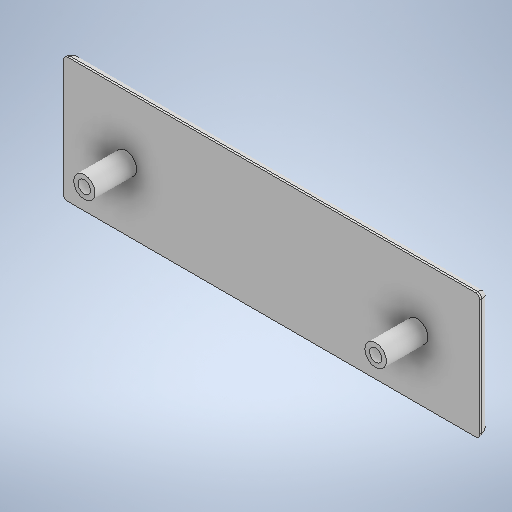
# Autodesk Inventor part: záslepka
Saved by Autodesk Inventor 2025 (Build 290162000, 162)
## iProperties
Created: 2025-01-12
Part Number: záslepka
Material: Všeobecné
Document SubType Name: Modeling
Designer: lukas
Density: 1 g/cm^3
Appearance: Výchozí
Author: lukas
## iProperties of the stored document záslepka_3D tisk.ipt
Created: 2025-01-18
Part Number: záslepka_3D tisk
Material: Všeobecné
Document SubType Name: Modeling
Designer: lukas
Density: 1 g/cm^3
Appearance: Výchozí
Author: lukas
Autodesk Inventor part; units mm, degrees
ref_plane "YZ Plane" through (0, 0, 0) normal (1, 0, 0) x (0, 1, 0)
ref_plane "XZ Plane" through (0, 0, 0) normal (0, 1, 0) x (-1, 0, 0)
ref_plane "XY Plane" through (0, 0, 0) normal (0, 0, 1) x (1, 0, 0)
sketch "Náčrt1" plane through (0, 0, 0) normal (0, 0, 1) x (1, 0, 0)
  line L0 (0, 21) -> (0, -21) projected
  line L1 (-70, 0) -> (70, 0) projected
  line L2 (-50, 15) -> (50, 15)
  line L3 (50, 15) -> (50, -15)
  line L4 (50, -15) -> (-50, -15)
  line L5 (-50, -15) -> (-50, 15)
  point P0 (0, 0)
  dimension "d0" = 100
  dimension "d1" = 30
  constraints: 8 end point, 2 parallel, 1 horizontal, 1 perpendicular, 2 other
  measures "d0" distance of L3.end L4.end
  measures "d1" distance of L2.end L3.end
extrude "Vysunutí1" add sketch "Náčrt1" along normal blind 2.5
sketch "Náčrt2" plane through (0, 0, 2.5) normal (0, 0, 1) x (1, 0, 0)
  line L0 (-50, -15) -> (50, -15) projected
  line L1 (50, -15) -> (50, 15) projected
  line L2 (50, 15) -> (-50, 15) projected
  line L3 (-50, 15) -> (-50, -15) projected
  line L4 (0, 21) -> (0, -21) projected
  line L5 (-70, 0) -> (70, 0) projected
  circle A0 centre (35, 0) radius 1.5
  circle A1 centre (35, 0) radius 2.575
  circle A2 centre (-35, 0) radius 1.5
  circle A3 centre (-35, 0) radius 2.575
  point P0 (0, 0)
  point P1 (50, 0)
  dimension "d11" = 3
  dimension "d12" = 5.15
  dimension "d13" = 15
  constraints: 4 centre point, 2 coincident, 2 symmetric about line, 1 midpoint, 1 point on line, 2 other
  measures "d11" diameter of A0
  measures "d12" diameter of A1
  measures "d13" distance of point (50, 0) A0.centre
fillet "Zaoblení1" radius 2 4 edges at (50, 0, 0) (0, 15, 0) (-50, 0, 0) (0, -15, 0)
fillet "Zaoblení2" radius 1 8 edges at (50, -15, 2.25) (49.4142, -14.4142, 0.5858) (50, 15, 2.25) (49.4142, 14.4142, 0.5858) (-50, 15, 2.25) (-49.4142, 14.4142, 0.5858) (-50, -15, 2.25) (-49.4142, -14.4142, 0.5858)
extrude "Vysunutí3" add sketch "Náčrt2" along normal blind 10 contours A3 L5 A2 | L5 A2 A3 | A1 L5 A0 | L5 A0 A1
